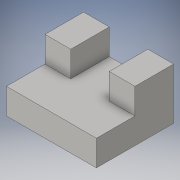
# Autodesk Inventor part: A2.6_Titus_SktechSheetA4
Saved by Autodesk Inventor 2016 (Build 200138000, 138)
## iProperties
Created: 2017-09-18
Part Number: A2.6_Titus_SktechSheetA4
Material: Generic
Document SubType Name: Modeling
Designer: sun01147
Density: 1 g/cm^3
Appearance: Default
Author: sun01147
Autodesk Inventor part; units mm, degrees
ref_plane "YZ Plane" through (0, 0, 0) normal (1, 0, 0) x (0, 1, 0)
ref_plane "XZ Plane" through (0, 0, 0) normal (0, 1, 0) x (-1, 0, 0)
ref_plane "XY Plane" through (0, 0, 0) normal (0, 0, 1) x (1, 0, 0)
sketch "Sketch1" plane through (0, 0, 0) normal (0, 0, 1) x (1, 0, 0)
  line L0 (0, 12.7) -> (44.45, 12.7)
  line L1 (44.45, 12.7) -> (44.45, 0)
  line L2 (44.45, 0) -> (0, 0)
  line L3 (0, 0) -> (0, 12.7)
  dimension "d0" = 44.45
  dimension "d1" = 12.7
  constraints: 8 end point, 2 parallel, 1 horizontal, 1 perpendicular
  measures "d0" distance of L1.end L2.end
  measures "d1" distance of L2.end L0.start
extrude "Extrusion1" add sketch "Sketch1" against normal blind 38.1
sketch "Sketch2" plane through (0, 12.7, 0) normal (0, 1, 0) x (1, 0, 0)
  line L0 (0, 0) -> (0, 38.1) projected
  line L1 (0, 38.1) -> (44.45, 38.1) projected
  line L2 (0, 19.05) -> (12.7, 19.05)
  line L3 (12.7, 19.05) -> (12.7, 38.1)
  line L4 (12.7, 38.1) -> (0, 38.1)
  line L5 (0, 38.1) -> (0, 19.05)
  line L6 (44.45, 0) -> (44.45, 38.1) projected
  line L7 (31.75, 38.1) -> (44.45, 38.1)
  line L8 (44.45, 38.1) -> (44.45, 19.05)
  line L9 (44.45, 19.05) -> (31.75, 19.05)
  line L10 (31.75, 19.05) -> (31.75, 38.1)
  dimension "d4" = 12.7
  dimension "d5" = 19.05
  dimension "d6" = 19.05
  dimension "d7" = 12.7
  constraints: 16 end point, 4 parallel, 2 horizontal, 2 midpoint, 2 perpendicular, 2 point on line
  measures "d4" distance of L2.start L2.end
  measures "d5" distance of L2.end L3.end
  measures "d6" distance of L9.end L7.start
  measures "d7" distance of L8.end L9.end
extrude "Extrusion2" add sketch "Sketch2" along normal blind 12.7
body "Solid1"
